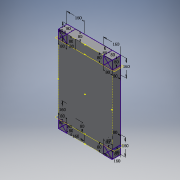
# Autodesk Inventor part: WireFrame
Saved by Autodesk Inventor 2018 (Build 220112000, 112)
## iProperties
Created: 2017-10-17
Part Number: WireFrame
Material: Generic
Document SubType Name: Modeling
Designer: Bryce Richards
Density: 1 g/cm^3
Appearance: Default
Mass: 32000 g
Surface Area: 10080 cm^2
Volume: 32000 cm^3
Author: Bryce Richards
Autodesk Inventor part; units mm, degrees
ref_plane "YZ Plane" through (0, 0, 0) normal (1, 0, 0) x (0, 1, 0)
ref_plane "XZ Plane" through (0, 0, 0) normal (0, 1, 0) x (-1, 0, 0)
ref_plane "XY Plane" through (0, 0, 0) normal (0, 0, 1) x (1, 0, 0)
sketch "Sketch1" plane through (0, 0, 0) normal (0, 1, 0) x (-1, 0, 0)
  line L0 (-250, 400) -> (250, 400)
  line L1 (250, 400) -> (250, -400)
  line L2 (250, -400) -> (-250, -400)
  line L3 (-250, -400) -> (-250, 400)
  line L4 (-250, 400) -> (250, -400) construction
  line L5 (250, 400) -> (-250, -400) construction
  point P0 (0, 0)
  dimension "d0" = 500
  dimension "d1" = 800
  constraints: 12 end point, 2 midpoint, 2 parallel, 1 horizontal, 1 perpendicular
  measures "d0" distance of L1.end L2.end
  measures "d1" distance of L0.end L1.end
extrude "Extrusion1" add sketch "Sketch1" along normal blind 80
sketch "Sketch2" plane through (0, 80, 0) normal (0, 1, 0) x (1, 0, 0)
  line L0 (-250, 400) -> (-250, -400) projected
  line L1 (-250, -400) -> (-250, 400)
  line L2 (250, 400) -> (-250, 400) projected
  line L3 (-250, 400) -> (250, 400)
  line L4 (250, -400) -> (250, 400) projected
  line L5 (250, 400) -> (250, -400)
  line L6 (-250, -400) -> (250, -400) projected
  line L7 (250, -400) -> (-250, -400)
  line L8 (170, 400) -> (170, 320)
  line L9 (170, 320) -> (250, 320)
  line L10 (250, -320) -> (170, -320)
  line L11 (170, -320) -> (170, -400)
  line L12 (-250, -320) -> (-170, -320)
  line L13 (-170, -320) -> (-170, -400)
  line L14 (-170, 400) -> (-170, 320)
  line L15 (-170, 320) -> (-250, 320)
  line L16 (-170, -320) -> (170, 320)
  line L17 (170, -320) -> (-170, 320)
  point P0 (0, 0)
  dimension "d21" = 80
  dimension "d22" = 80
  dimension "d23" = 80
  dimension "d24" = 80
  dimension "d25" = 80
  dimension "d26" = 80
  dimension "d27" = 80
  constraints: 28 end point, 10 point on line, 7 perpendicular, 4 collinear
  measures "d21" distance of L8.start L8.end
  measures "d22" distance of L8.end L9.end
  measures "d23" distance of L10.start L10.end
  measures "d24" distance of L10.end L11.end
  measures "d25" distance of L12.end L13.end
  measures "d26" distance of L12.start L12.end
  measures "d27" distance of L14.start L14.end
sketch "Sketch3" plane through (0, 0, 0) normal (0, -1, 0) x (1, 0, 0)
  line L0 (250, 400) -> (170, 400)
  line L1 (170, 400) -> (170, 320)
  line L2 (170, 320) -> (250, 320)
  line L3 (250, 320) -> (250, 400)
  line L4 (250, -400) -> (170, -400)
  line L5 (170, -400) -> (170, -320)
  line L6 (170, -320) -> (250, -320)
  line L7 (250, -320) -> (250, -400)
  line L8 (-250, 400) -> (-170, 400)
  line L9 (-170, 400) -> (-170, 320)
  line L10 (-170, 320) -> (-250, 320)
  line L11 (-250, 320) -> (-250, 400)
  line L12 (-250, -400) -> (-170, -400)
  line L13 (-170, -400) -> (-170, -320)
  line L14 (-170, -320) -> (-250, -320)
  line L15 (-250, -320) -> (-250, -400)
  line L16 (170, 320) -> (250, 400)
  line L17 (170, 400) -> (250, 320)
  line L18 (-170, 320) -> (-250, 400)
  line L19 (-170, 400) -> (-250, 320)
  line L20 (-170, -320) -> (-250, -400)
  line L21 (-170, -400) -> (-250, -320)
  line L22 (170, -320) -> (250, -400)
  line L23 (170, -400) -> (250, -320)
  point P0 (0, 0)
  dimension "d4" = 80
  dimension "d5" = 80
  dimension "d6" = 80
  dimension "d7" = 80
  dimension "d8" = 80
  dimension "d9" = 80
  dimension "d10" = 80
  dimension "d11" = 80
  constraints: 48 end point, 8 parallel, 5 perpendicular, 4 horizontal
  measures "d4" distance of L2.end L1.end
  measures "d5" distance of L1.end L0.end
  measures "d6" distance of L5.end L6.end
  measures "d7" distance of L4.end L5.end
  measures "d8" distance of L9.end L10.end
  measures "d9" distance of L8.end L9.end
  measures "d10" distance of L14.end L13.end
  measures "d11" distance of L13.end L12.end
sketch "Sketch4" plane through (-250, 0, 400) normal (0, 0, 1) x (1, 0, 0)
  line L0 (0, 80) -> (500, 80) projected
  line L1 (0, 0) -> (0, 80) projected
  line L2 (0, 80) -> (0, 0)
  line L3 (500, 80) -> (500, 0)
  line L4 (500, 0) -> (500, 80) projected
  line L5 (80, 80) -> (80, 0)
  line L6 (420, 0) -> (420, 80)
  point P0 (250, 0)
  dimension "d13" = 80
  dimension "d14" = 80
  dimension "d42" = 80
  dimension "d43" = 80
  constraints: 8 end point, 2 point on line, 2 vertical, 1 perpendicular
  measures "d13" distance between parallel lines of L1 L5
  measures "d14" distance between parallel lines of L3 L6
  measures "d42" distance from line of L6.start L0
  measures "d43" distance from line of L5.end L0
sketch "Sketch5" plane through (250, 0, -400) normal (0, 0, -1) x (-1, 0, 0)
  line L0 (500, 80) -> (0, 80) projected
  line L1 (0, 80) -> (0, 0)
  line L2 (500, 0) -> (500, 80) projected
  line L3 (500, 80) -> (500, 0)
  line L4 (80, 80) -> (80, 0)
  line L5 (420, 80) -> (420, 0)
  point P0 (250, 0)
  dimension "d15" = 80
  dimension "d16" = 80
  dimension "d44" = 80
  dimension "d45" = 80
  constraints: 8 end point, 3 vertical, 2 point on line
  measures "d15" distance between parallel lines of L1 L4
  measures "d16" distance between parallel lines of L2 L5
  measures "d44" distance from line of L5.end L0
  measures "d45" distance from line of L4.end L0
sketch "Sketch6" plane through (250, 0, 400) normal (1, 0, 0) x (0, 0, -1)
  line L0 (80, 0) -> (80, 79.4534)
  line L1 (720, -0.5466) -> (720, 79.4534)
  line L2 (800, 0) -> (800, 80) projected
  line L3 (0, 0) -> (0, 80) projected
  point P0 (400, 0)
  dimension "d17" = 80
  dimension "d18" = 80
  dimension "d41" = 80
  constraints: 4 end point, 2 vertical
  measures "d17" distance between parallel lines of L2 L1
  measures "d18" distance between parallel lines of L3 L0
  measures "d41" distance of L1.start L1.end
sketch "Sketch7" plane through (-250, 0, -400) normal (-1, 0, 0) x (0, 0, 1)
  line L0 (800, 80) -> (0, 80) projected
  line L1 (80, 80) -> (80, 0)
  line L2 (720, 80) -> (720, 0)
  line L3 (0, 0) -> (0, 80) projected
  line L4 (800, 0) -> (800, 80) projected
  point P0 (400, 0)
  dimension "d19" = 80
  dimension "d20" = 80
  constraints: 4 end point, 2 point on line, 2 vertical
  measures "d19" distance between parallel lines of L3 L1
  measures "d20" distance between parallel lines of L4 L2
sketch "Sketch9" plane through (-250, 0, 400) normal (0, 0, 1) x (1, 0, 0)
  line L0 (0, 80) -> (500, 80) construction
  line L1 (0, 0) -> (0, 80) construction
  line L2 (500, 0) -> (500, 80) construction
  line L3 (0, 0) -> (0, 80) construction
  line L4 (0, 80) -> (0, 0) construction
  line L5 (500, 0) -> (500, 80) construction
  point P0 (250, 0)
  constraints: 4 end point, 1 parallel
ref_plane "Work Plane1" through (-250, 0, 320) normal (0, 0, 1) x (1, 0, 0)
ref_plane "Work Plane2" through (250, 0, -320) normal (0, 0, -1) x (-1, 0, 0)
sketch "Sketch10" plane through (-250, 0, 320) normal (0, 0, 1) x (1, 0, 0)
  line L0 (80, 80) -> (80, 0) construction
  line L1 (420, 0) -> (420, 80) construction
  line L2 (80, 80) -> (80, 0)
  line L3 (420, 80) -> (420, 0)
  point P0 (250, 0)
  constraints: 4 end point, 2 collinear
sketch "Sketch11" plane through (250, 0, -320) normal (0, 0, -1) x (-1, 0, 0)
  line L0 (80, 80) -> (80, 0) construction
  line L1 (420, 80) -> (420, 0) construction
  line L2 (80, 80) -> (80, 0)
  line L3 (420, 80) -> (420, 0)
  point P0 (250, 0)
  constraints: 4 end point, 1 collinear, 1 vertical
body "Solid1"
